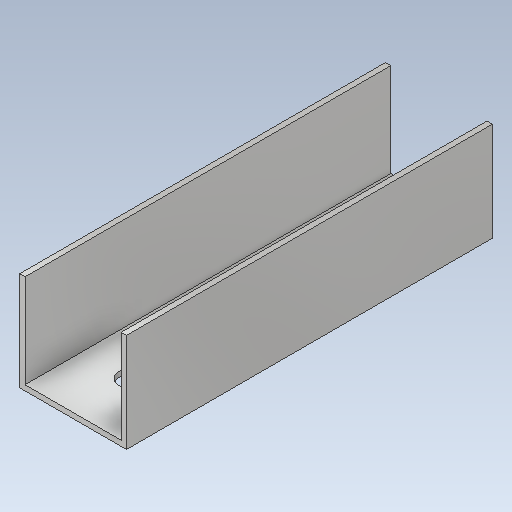
# Autodesk Inventor part: motor_base
Saved by Autodesk Inventor 2020 (Build 240168000, 168)
## iProperties
Created: 2017-11-25
Part Number: motor_base
Material: Generic
Document SubType Name: Modeling
Designer: stedrock
Density: 1 g/cm^3
Appearance: Default
Mass: 29.8977 g
Surface Area: 309.957 cm^2
Volume: 29.8977 cm^3
Author: stedrock
Autodesk Inventor part; units mm, degrees
ref_plane "YZ Plane" through (0, 0, 0) normal (1, 0, 0) x (0, 1, 0)
ref_plane "XZ Plane" through (0, 0, 0) normal (0, 1, 0) x (-1, 0, 0)
ref_plane "XY Plane" through (0, 0, 0) normal (0, 0, 1) x (1, 0, 0)
sketch "Sketch1" plane through (0, 0, 0) normal (0, 0, 1) x (1, 0, 0)
  line L0 (-20, 20) -> (20, 20)
  line L1 (20, 20) -> (20, -20)
  line L2 (20, -20) -> (-20, -20)
  line L3 (-20, -20) -> (-20, 20)
  line L4 (-20, 20) -> (20, -20) construction
  line L5 (20, 20) -> (-20, -20) construction
  line L6 (-18, -18) -> (18, -18)
  line L7 (18, -18) -> (18, 18)
  line L8 (18, 18) -> (-18, 18)
  line L9 (-18, 18) -> (-18, -18)
  line L10 (-18, -18) -> (18, 18) construction
  line L11 (18, -18) -> (-18, 18) construction
  line L12 (-20, 20) -> (20, 20)
  line L13 (20, 20) -> (20, 17)
  line L14 (20, 17) -> (-20, 17)
  line L15 (-20, 17) -> (-20, 20)
  point P0 (0, 0)
  dimension "d0" = 40
  dimension "d1" = 40
  dimension "d2" = 36
  dimension "d3" = 36
  dimension "d6" = 35
  constraints: 32 end point, 6 parallel, 4 midpoint, 3 horizontal, 3 perpendicular, 1 point on line
  measures "d0" distance of L1.end L2.end
  measures "d1" distance of L0.end L1.end
  measures "d2" distance of L8.end L7.end
  measures "d3" distance of L7.end L6.end
  measures "d6" distance between parallel lines of L6 L14
extrude "Extrusion2" add sketch "Sketch1" along normal blind 137 contours L14 L9 L6 L7 L1 L2 L3
sketch "Sketch2" plane through (-20, -20, 0) normal (0, -1, 0) x (1, 0, 0)
  circle A0 centre (20, 80) radius 4
  line L0 (20, 0) -> (20, 151.5414) construction
  circle A1 centre (20, 115) radius 4.75
  line L1 (0, 0) -> (40, 0) projected
  dimension "d9" = 8
  dimension "d11" = 9.5
  dimension "d12" = 80
  dimension "d15" = 35
  constraints: 2 centre point, 2 end point, 2 point on line, 1 vertical
  measures "d9" diameter of A0
  measures "d11" diameter of A1
  measures "d12" distance from line of L1 A0.centre
  measures "d15" distance of A0.centre A1.centre
extrude "Extrusion3" cut sketch "Sketch2" against normal through all
body "Solid2"
